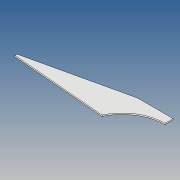
# Autodesk Inventor part: Center_fin
Saved by Autodesk Inventor 2019.4 (Build 234330000, 330)
## iProperties
Part Number: Center_fin
Material: GEDA Polyamid
Document SubType Name: Modeling
Designer: Admin
Mass: 45.4902 g
Surface Area: 287.49 cm^2
Volume: 39.9037 cm^3
Density: 1.14 g/cm^3
Appearance: GEDA Polyamid A
Gewicht: 0,045 kg
G_L: 0
G_H: 0
G_B: 0
InventorVersion: 2019.4
VAULT_Status: in Bearbeitung
Revision: -
Max. Breite: 0
Max. Höhe: 0
Max. Länge: 0
Max. Abmessungen: 0 x 0 x 0
Author: Admin
Autodesk Inventor part; units mm, degrees
note: some values were not read from the file. Left out: dimensions or parameters whose unit could not be read.
ref_plane "YZ Plane" through (0, 0, 0) normal (1, 0, 0) x (0, 1, 0)
ref_plane "XZ Plane" through (0, 0, 0) normal (0, 1, 0) x (-1, 0, 0)
ref_plane "XY Plane" through (0, 0, 0) normal (0, 0, 1) x (1, 0, 0)
sketch "Skizze1" plane through (0, 0, 0) normal (0, 0, 1) x (1, 0, 0)
  line L0 (-71, 0) -> (391, 0) projected
  line L1 (-5, 35) -> (-5, 30)
  line L2 (-5, 30) -> (229.7825, 10)
  line L3 (325, 70) -> (325, 110)
  line L4 (325, 110) -> (-5, 35)
  arc A0 (325, 70) -> (229.7825, 10) centre (325, -35.5531) ccw
  line L5 (325, 90) -> (237, 90)
  point P0 (0, 0)
  dimension "d3" = 5
  dimension "d5" = 330
  dimension "d6" = 40
  dimension "d7" = 5
  dimension "d8" = 30
  dimension "d9" = 230
  dimension "d13" = 10
  dimension "d14" = 70
  constraints: 10 end point, 2 point on circle, 1 centre point, 1 horizontal, 1 line through centre, 1 midpoint, 1 parallel, 1 point on line, 1 vertical
  measures "d3" distance of L1.start L1.end
  measures "d5" distance between parallel lines of L3 L1
  measures "d6" distance of L3.start L3.end
  measures "d7" distance from line of point (0, 0) L1
  measures "d8" distance from line of L0 L1.end
  measures "d9" distance of L2.end point (0, 0)
  measures "d13" distance from line of L0 L2.end
  measures "d14" distance from line of L0 L3.start
extrude "Extrusion1" add sketch "Skizze1" along normal blind 3 contours L4 L5 L3 A0 L2 L1
equation "\"G_L\" = 0"
equation "\"G_H\" = 0"
equation "\"G_B\" = 0"
